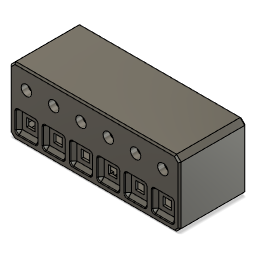
Deej oxivanisher remix v3 (Autodesk Fusion 360 design; units mm, degrees)
Autodesk Fusion 360 part; units mm, degrees
sketch "Sketch1" plane through (0, 0, 0) normal (0, 0, 1) x (1, 0, 0)
  circle A0 centre (0, 0) radius 3.45
  line L0 (9, -30) -> (-9, -30)
  line L1 (-9, -30) -> (-9, 10)
  line L2 (-9, 10) -> (9, 10)
  line L3 (9, 10) -> (9, -30)
  line L4 (9, -30) -> (-9, 10) construction
  line L5 (-9, -30) -> (9, 10) construction
  line L6 (0, 10) -> (0, -30) construction
  line L7 (-9, 1.45) -> (-6, 1.45)
  line L8 (-6, 1.45) -> (-6, -1.45)
  line L9 (-6, -1.45) -> (-9, -1.45)
  line L10 (-6, 0) -> (0, 0) construction
  line L11 (-9, -12) -> (9, -12) construction
  line L12 (-9, -30) -> (9, -12) construction
  line L13 (2.75, -23.75) -> (-2.75, -23.75)
  line L14 (-2.75, -23.75) -> (-2.75, -18.25)
  line L15 (-2.75, -18.25) -> (2.75, -18.25)
  line L16 (2.75, -18.25) -> (2.75, -23.75)
  line L17 (2.75, -23.75) -> (-2.75, -18.25) construction
  line L18 (-2.75, -23.75) -> (2.75, -18.25) construction
  line L19 (7.6, -28.6) -> (-7.6, -28.6)
  line L20 (-7.6, -28.6) -> (-7.6, -13.4)
  line L21 (-7.6, -13.4) -> (7.6, -13.4)
  line L22 (7.6, -13.4) -> (7.6, -28.6)
  line L23 (7.6, -28.6) -> (-7.6, -13.4) construction
  line L24 (-7.6, -28.6) -> (7.6, -13.4) construction
  point P0 (0, -10)
  point P1 (0, -21)
  point P2 (0, -21)
  point P3 (0, -21)
  dimension "d1" = 6.9
  dimension "d2" = 18
  dimension "d3" = 40
  dimension "d4" = 10
  dimension "d5" = 2.9
  dimension "d6" = 3
  dimension "d7" = 18
  dimension "d8" = 5.5
  dimension "d9" = 5.5
  dimension "d10" = 15.2
  dimension "d11" = 15.2
  constraint coincident A0.centre L10.end
  constraint horizontal L0
  constraint perpendicular L0 L1
  constraint parallel L0 L2
  constraint parallel L1 L3
  constraint coincident L4 P0
  constraint coincident L5 P0
  constraint midpoint L2 L6.start
  constraint midpoint L0 L6.end
  constraint coincident A0.centre L6
  constraint coincident L1 L7.start
  constraint perpendicular L1 L7
  constraint perpendicular L7 L8
  constraint coincident L1 L9.end
  constraint perpendicular L1 L9
  constraint midpoint L8 L10.start
  constraint horizontal L10
  constraint coincident L1 L11.start
  constraint coincident L3 L11.end
  constraint perpendicular L3 L11
  constraint midpoint L12 P3
  constraint horizontal L13
  constraint perpendicular L13 L14
  constraint parallel L13 L15
  constraint parallel L14 L16
  constraint coincident L17 P3
  constraint coincident L18 P3
  constraint coincident P3 P2
  constraint horizontal L19
  constraint perpendicular L19 L20
  constraint parallel L19 L21
  constraint parallel L20 L22
  constraint coincident L23 P3
  constraint coincident L24 P3
  measures "d1" diameter of A0
  measures "d2" distance of L1.end L2.end
  measures "d3" distance of L0.end L1.end
  measures "d4" distance of A0.centre L2
  measures "d5" distance of L7.end L8.end
  measures "d6" distance of L7.start L7.end
  measures "d7" distance of L0 L11
  measures "d8" distance of L14.end L15.end
  measures "d9" distance of L13.end L14.end
  measures "d10" distance of L20.end L21.end
  measures "d11" distance of L19.end L20.end
extrude "Extrude1" add sketch "Sketch1" along normal blind 1.4 contours L0 L1 L2 L3 L7 L8 L9 | L1 L7 L8 L9 makes body 1
extrude "Extrude2" add sketch "Sketch1" against normal blind 1.5 contours L0 L1 L2 L3 L7 L8 L9 bodies 1
sketch "Sketch2" plane through (0, 0, -1.5) normal (0, 0, -1) x (-1, 0, 0)
  circle A0 centre (0, 0) radius 3.45
  line L0 (-7.6, -13.4) -> (7.6, -13.4)
  line L1 (7.6, -13.4) -> (7.6, -28.6)
  line L2 (7.6, -28.6) -> (-7.6, -28.6)
  line L3 (-7.6, -28.6) -> (-7.6, -13.4)
  line L4 (6, 1.45) -> (9, 1.45)
  line L5 (9, 1.45) -> (9, 10)
  line L6 (9, 10) -> (-9, 10)
  line L7 (-9, 10) -> (-9, -30)
  line L8 (-9, -30) -> (9, -30)
  line L9 (9, -30) -> (9, -1.45)
  line L10 (9, -1.45) -> (6, -1.45)
  line L11 (6, -1.45) -> (6, 1.45)
  line L12 (2.75, -18.25) -> (-2.75, -18.25)
  line L13 (2.75, -23.75) -> (2.75, -18.25)
  line L14 (-2.75, -23.75) -> (2.75, -23.75)
  line L15 (-2.75, -18.25) -> (-2.75, -23.75)
extrude "Extrude3" add sketch "Sketch2" along normal blind 1.4 contours L0 L1 L2 L3 | L4 L5 L6 L7 L8 L9 L10 L11 bodies 1
fillet "Fillet1" radius 2 4 edges at (7.6, -13.4, -0.05) (-7.6, -13.4, -0.05) (7.6, -28.6, -0.05) (-7.6, -28.6, -0.05) on bodies 1
chamfer "Chamfer1" distance 2 angle 45 8 edges at (7.0142, -13.9858, -1.5) (0, -13.4, -1.5) (-7.0142, -13.9858, -1.5) (-7.6, -21, -1.5) (-7.0142, -28.0142, -1.5) (0, -28.6, -1.5) (7.0142, -28.0142, -1.5) (7.6, -21, -1.5) on bodies 1
pattern_linear "R-Pattern1" count 6 spacing 18 along (1, 0, 0) of bodies 1 makes body 2 at (11.0833, -16.5667, -2.9) makes body 3 at (29.0833, -16.5667, -2.9) makes body 4 at (47.0833, -16.5667, -2.9) makes body 5 at (65.0833, -16.5667, -2.9) makes body 6 at (83.0833, -16.5667, -2.9)
combine "Combine1" operation add target body 1 tool bodies 3 2 4 6 5
sketch "Sketch3" plane through (0, 0, 1.4) normal (0, 0, 1) x (1, 0, 0)
  circle A0 centre (90, 0) radius 3.45
  line L0 (84.4, -13.4) -> (95.6, -13.4)
  arc A1 (97.6, -15.4) -> (95.6, -13.4) centre (95.6, -15.4) ccw
  line L1 (97.6, -15.4) -> (97.6, -26.6)
  arc A2 (95.6, -28.6) -> (97.6, -26.6) centre (95.6, -26.6) ccw
  line L2 (95.6, -28.6) -> (84.4, -28.6)
  arc A3 (82.4, -26.6) -> (84.4, -28.6) centre (84.4, -26.6) ccw
  line L3 (82.4, -26.6) -> (82.4, -15.4)
  arc A4 (84.4, -13.4) -> (82.4, -15.4) centre (84.4, -15.4) ccw
  line L4 (66.4, -13.4) -> (77.6, -13.4)
  arc A5 (79.6, -15.4) -> (77.6, -13.4) centre (77.6, -15.4) ccw
  line L5 (79.6, -15.4) -> (79.6, -26.6)
  arc A6 (77.6, -28.6) -> (79.6, -26.6) centre (77.6, -26.6) ccw
  line L6 (77.6, -28.6) -> (66.4, -28.6)
  arc A7 (64.4, -26.6) -> (66.4, -28.6) centre (66.4, -26.6) ccw
  line L7 (64.4, -26.6) -> (64.4, -15.4)
  arc A8 (66.4, -13.4) -> (64.4, -15.4) centre (66.4, -15.4) ccw
  circle A9 centre (72, 0) radius 3.45
  circle A10 centre (54, 0) radius 3.45
  line L8 (48.4, -13.4) -> (59.6, -13.4)
  arc A11 (61.6, -15.4) -> (59.6, -13.4) centre (59.6, -15.4) ccw
  line L9 (61.6, -15.4) -> (61.6, -26.6)
  arc A12 (59.6, -28.6) -> (61.6, -26.6) centre (59.6, -26.6) ccw
  line L10 (59.6, -28.6) -> (48.4, -28.6)
  arc A13 (46.4, -26.6) -> (48.4, -28.6) centre (48.4, -26.6) ccw
  line L11 (46.4, -26.6) -> (46.4, -15.4)
  arc A14 (48.4, -13.4) -> (46.4, -15.4) centre (48.4, -15.4) ccw
  circle A15 centre (36, 0) radius 3.45
  line L12 (30.4, -13.4) -> (41.6, -13.4)
  arc A16 (43.6, -15.4) -> (41.6, -13.4) centre (41.6, -15.4) ccw
  line L13 (43.6, -15.4) -> (43.6, -26.6)
  arc A17 (41.6, -28.6) -> (43.6, -26.6) centre (41.6, -26.6) ccw
  line L14 (41.6, -28.6) -> (30.4, -28.6)
  arc A18 (28.4, -26.6) -> (30.4, -28.6) centre (30.4, -26.6) ccw
  line L15 (28.4, -26.6) -> (28.4, -15.4)
  arc A19 (30.4, -13.4) -> (28.4, -15.4) centre (30.4, -15.4) ccw
  line L16 (12.4, -13.4) -> (23.6, -13.4)
  arc A20 (25.6, -15.4) -> (23.6, -13.4) centre (23.6, -15.4) ccw
  line L17 (25.6, -15.4) -> (25.6, -26.6)
  arc A21 (23.6, -28.6) -> (25.6, -26.6) centre (23.6, -26.6) ccw
  line L18 (23.6, -28.6) -> (12.4, -28.6)
  arc A22 (10.4, -26.6) -> (12.4, -28.6) centre (12.4, -26.6) ccw
  line L19 (10.4, -26.6) -> (10.4, -15.4)
  arc A23 (12.4, -13.4) -> (10.4, -15.4) centre (12.4, -15.4) ccw
  circle A24 centre (18, 0) radius 3.45
  line L20 (-5.6, -13.4) -> (5.6, -13.4)
  arc A25 (7.6, -15.4) -> (5.6, -13.4) centre (5.6, -15.4) ccw
  line L21 (7.6, -15.4) -> (7.6, -26.6)
  arc A26 (5.6, -28.6) -> (7.6, -26.6) centre (5.6, -26.6) ccw
  line L22 (5.6, -28.6) -> (-5.6, -28.6)
  arc A27 (-7.6, -26.6) -> (-5.6, -28.6) centre (-5.6, -26.6) ccw
  line L23 (-7.6, -26.6) -> (-7.6, -15.4)
  arc A28 (-5.6, -13.4) -> (-7.6, -15.4) centre (-5.6, -15.4) ccw
  circle A29 centre (0, 0) radius 3.45
  line L24 (99, 10) -> (-9, 10)
  line L25 (-9, 10) -> (-9, -30)
  line L26 (-9, -30) -> (99, -30)
  line L27 (99, -30) -> (99, 10)
  line L28 (-11, -32) -> (101, -32)
  line L29 (101, -32) -> (101, 12)
  line L30 (101, 12) -> (-11, 12)
  line L31 (-11, 12) -> (-11, -32)
  dimension "d25" = 2
extrude "Extrude4" add sketch "Sketch3" against normal blind 44 contours L28 L29 L30 L31 bodies 1
chamfer "Chamfer2" distance 2 angle 45 4 edges at (-9, 10, -22.75) (99, 10, -22.75) (99, -30, -22.75) (-9, -30, -22.75) on bodies 1
chamfer "Chamfer3" distance 3 angle 45 4 edges at (-11, 12, -20.6) (-11, -32, -20.6) (101, 12, -20.6) (101, -32, -20.6) on bodies 1
chamfer "Chamfer4" distance 1 angle 45 16 edges at (45, 12, 1.4) (-9.5, 10.5, 1.4) (-11, -10, 1.4) (-9.5, -30.5, 1.4) (45, -32, 1.4) (99.5, 10.5, 1.4) (101, -10, 1.4) (99.5, -30.5, 1.4) (101, -10, -42.6) (99.5, 10.5, -42.6) (45, 12, -42.6) (99.5, -30.5, -42.6) (45, -32, -42.6) (-9.5, -30.5, -42.6) (-11, -10, -42.6) (-9.5, 10.5, -42.6) on bodies 1
sketch "Sketch4" plane through (0, 0, -42.6) normal (0, 0, -1) x (-1, 0, 0)
  line L0 (-99, -28) -> (-99, 8)
  line L1 (-99, 8) -> (-97, 10)
  line L2 (-97, 10) -> (7, 10)
  line L3 (7, 10) -> (9, 8)
  line L4 (9, 8) -> (9, -28)
  line L5 (9, -28) -> (7, -30)
  line L6 (7, -30) -> (-97, -30)
  line L7 (-97, -30) -> (-99, -28)
  line L8 (10, -28.5858) -> (10, 8.5858)
  line L9 (10, 8.5858) -> (7.5858, 11)
  line L10 (7.5858, 11) -> (-97.5858, 11)
  line L11 (-97.5858, 11) -> (-100, 8.5858)
  line L12 (-100, 8.5858) -> (-100, -28.5858)
  line L13 (-100, -28.5858) -> (-97.5858, -31)
  line L14 (-97.5858, -31) -> (7.5858, -31)
  line L15 (7.5858, -31) -> (10, -28.5858)
  line L16 (8.8, 7.9172) -> (8.8, -27.9172)
  line L17 (8.8, -27.9172) -> (6.9172, -29.8)
  line L18 (6.9172, -29.8) -> (-96.9172, -29.8)
  line L19 (-96.9172, -29.8) -> (-98.8, -27.9172)
  line L20 (-98.8, -27.9172) -> (-98.8, 7.9172)
  line L21 (-98.8, 7.9172) -> (-96.9172, 9.8)
  line L22 (-96.9172, 9.8) -> (6.9172, 9.8)
  line L23 (6.9172, 9.8) -> (8.8, 7.9172)
  circle A0 centre (-95.8, 6.8) radius 3 construction
  circle A1 centre (-95.8, -26.8) radius 3 construction
  circle A2 centre (5.8, -26.8) radius 3 construction
  circle A3 centre (5.8, 6.8) radius 3 construction
  circle A4 centre (-95.8, 6.8) radius 1.6
  circle A5 centre (-95.8, -26.8) radius 1.6
  circle A6 centre (5.8, -26.8) radius 1.6
  circle A7 centre (5.8, 6.8) radius 1.6
  line L24 (-49, -23.3) -> (-41, -23.3)
  line L25 (-41, -23.3) -> (-41, -26.3)
  line L26 (-41, -26.3) -> (-49, -26.3)
  line L27 (-49, -26.3) -> (-49, -23.3)
  line L28 (-41, -29.8) -> (-41, -27.8)
  line L29 (-41, -27.8) -> (-49, -27.8)
  line L30 (-49, -27.8) -> (-49, -29.8)
  line L31 (-45, -27.8) -> (-45, -26.3) construction
  line L32 (-45, -29.8) -> (-45, -27.8) construction
  line L33 (-99, -0.4853) -> (-88.5147, 10)
  line L34 (-1.4853, 10) -> (9, -0.4853)
  line L35 (9, -19.5147) -> (-1.4853, -30)
  line L36 (-88.5147, -30) -> (-99, -19.5147)
  circle A8 centre (-95.8, 6.8) radius 1.5
  circle A9 centre (5.8, 6.8) radius 1.5
  circle A10 centre (5.8, -26.8) radius 1.5
  circle A11 centre (-95.8, -26.8) radius 1.5
  line L37 (-49, -27.8) -> (-49, -26.3)
  line L38 (-41, -27.8) -> (-41, -26.3)
  line L39 (-49, -28.8) -> (-41, -28.8)
  point P0 (-45, -29.8)
  dimension "d35" = 0.2
  dimension "d36" = 6
  dimension "d37" = 6
  dimension "d38" = 6
  dimension "d39" = 6
  dimension "d40" = 3.2
  dimension "d41" = 3.2
  dimension "d42" = 3.2
  dimension "d43" = 3.2
  dimension "d44" = 8
  dimension "d45" = 3
  dimension "d46" = 2
  dimension "d47" = 1.5
  dimension "d54" = 6
  dimension "d55" = 6
  dimension "d56" = 6
  dimension "d57" = 6
  dimension "d58" = 3
  dimension "d59" = 3
  dimension "d60" = 3
  dimension "d61" = 3
  constraint tangent L22 A0
  constraint tangent L20 A0
  constraint tangent L20 A1
  constraint tangent L18 A1
  constraint tangent L22 A3
  constraint tangent L16 A3
  constraint tangent L16 A2
  constraint tangent L18 A2
  constraint concentric A0 A4
  constraint concentric A1 A5
  constraint concentric A2 A6
  constraint concentric A3 A7
  constraint midpoint L18 P0
  constraint horizontal L24
  constraint vertical L25
  constraint horizontal L26
  constraint vertical L27
  constraint coincident L18 L28.start
  constraint perpendicular L18 L28
  constraint perpendicular L25 L29
  constraint coincident L18 L30.end
  constraint perpendicular L18 L30
  constraint midpoint L29 L31.start
  constraint midpoint L26 L31.end
  constraint perpendicular L26 L31
  constraint coincident P0 L32.start
  constraint vertical L32
  constraint collinear L27 L30
  constraint coincident L0 L33.start
  constraint coincident L2 L33.end
  constraint parallel L1 L33
  constraint coincident L2 L34.start
  constraint coincident L4 L34.end
  constraint parallel L3 L34
  constraint coincident L4 L35.start
  constraint coincident L6 L35.end
  constraint parallel L5 L35
  constraint coincident L6 L36.start
  constraint coincident L0 L36.end
  constraint parallel L7 L36
  constraint concentric A0 A8
  constraint concentric A3 A9
  constraint concentric A2 A10
  constraint concentric A1 A11
  constraint midpoint L30 L39.start
  constraint midpoint L28 L39.end
  measures "d36" diameter of A0
  measures "d37" diameter of A1
  measures "d38" diameter of A2
  measures "d39" diameter of A3
  measures "d40" diameter of A4
  measures "d41" diameter of A5
  measures "d42" diameter of A6
  measures "d43" diameter of A7
  measures "d44" distance of L24.start L24.end
  measures "d45" distance of L24.start L26.end
  measures "d46" distance of L28.start L28.end
  measures "d47" distance of L31.start L31.end
  measures "d54" distance of L1 L33
  measures "d55" distance of L3 L34
  measures "d56" distance of L5 L35
  measures "d57" distance of L7 L36
  measures "d58" diameter of A8
  measures "d59" diameter of A9
  measures "d60" diameter of A10
  measures "d61" diameter of A11
extrude "Extrude5" add sketch "Sketch4" against normal blind 1.4 separate body contours L18 L19 L20 L36 | L16 L18 L20 L22 L24 L25 L27 L28 L30 L33 L34 L35 L36 L37 L38 | L20 L21 L22 L33 | L18 L28 L30 L39 | L16 L17 L18 L35 | L16 L22 L23 L34 | L28 L29 L30 L39 | L26 L29 L37 L38 makes body 7
extrude "Extrude6" add sketch "Sketch4" against normal up to surface (38.3 mm away) from surface at -1.4 contours L18 L28 L30 L39 bodies 1
extrude "Extrude7" add sketch "Sketch4" against normal blind 20 from surface at -1.4 contours L0 L6 L7 L18 L19 L20 L36 | L0 L1 L2 L20 L21 L22 L33 | L18 L19 L20 L36 | L20 L21 L22 L33 | L4 L5 L6 L16 L17 L18 L35 | L16 L17 L18 L35 | L2 L3 L4 L16 L22 L23 L34 | L16 L22 L23 L34 | A4 | A5 | A6 | A7 bodies 1
chamfer "Chamfer5" distance 6 distance2 15 4 edges at (93.7574, 4.7574, -21.2) (93.7574, -24.7574, -21.2) (-3.7574, 4.7574, -21.2) (-3.7574, -24.7574, -21.2) measured on face at (93.5216, 9.3663, -21.2) measured on face at (93.5216, -29.3663, -21.2) measured on face at (-3.5216, 9.3663, -21.2) measured on face at (-3.5216, -29.3663, -21.2) on bodies 1
extrude "Extrude8" add sketch "Sketch4" against normal up to surface (4.3 mm away) from surface at -35.4 contours L28 L29 L30 L39 | L26 L29 L37 L38 bodies 1
hidden bodies 7
equation "d67 = -( 1.4 mm + 34 mm )"
named bodies: "Deej oXiVanisher Remix Case", "Deej oXiVanisher Remix Lid (1)", "Deej oXiVanisher Remix Lid (2)", "Deej oXiVanisher Remix Lid (3)", "Deej oXiVanisher Remix Lid (4)", "Deej oXiVanisher Remix Lid (5)", "Deej oXiVanisher Remix Lid"
